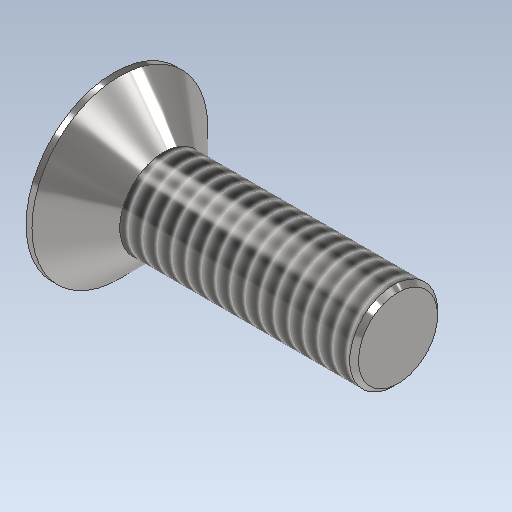
# Autodesk Inventor part: ネジ皿M3L8
Saved by Autodesk Inventor 2020.2 (Build 242310000, 310)
## iProperties
Created: 2020-04-20
Part Number: ネジ皿M3L8
Material: 鋼、高強度、低合金
Document SubType Name: Modeling
Designer: aoyama
Density: 7.85 g/cm^3
Appearance: 鋼 - つや出し
Mass: 0.649002 g
Surface Area: 1.51758 cm^2
Volume: 0.0826754 cm^3
Author: aoyama
Autodesk Inventor part; units mm, degrees
ref_plane "YZ Plane" through (0, 0, 0) normal (1, 0, 0) x (0, 1, 0)
ref_plane "XZ Plane" through (0, 0, 0) normal (0, 1, 0) x (-1, 0, 0)
ref_plane "XY Plane" through (0, 0, 0) normal (0, 0, 1) x (1, 0, 0)
sketch "スケッチ1" plane through (0, 0, 0) normal (0, 0, 1) x (1, 0, 0)
  line L0 (0, 0) -> (0, 3)
  line L1 (0, 3) -> (0.2, 3)
  line L2 (0.2, 3) -> (1.7, 1.5)
  line L3 (1.7, 1.5) -> (9.7, 1.5)
  line L4 (9.7, 1.5) -> (9.7, 0)
  line L5 (0, 0) -> (9.7, 0)
  dimension "d0" = 45
  dimension "d1" = 3
  dimension "d2" = 1.7
  dimension "d3" = 1.5
  dimension "d4" = 8
  constraints: 12 end point, 3 horizontal, 2 vertical
  measures "d0" angle of L0 L2
  measures "d1" distance of L0.start L0.end
  measures "d2" distance from line of L0 L2.end
  measures "d3" distance between parallel lines of L3 L5
  measures "d4" distance of L3.end L2.end
revolve "回転1" add sketch "スケッチ1" angle 360 about axis through (0, 0, 0) along (1, 0, 0)
thread "ねじ1" size "M3x0.5" class "6g" standard "ANSI Metric M Profile" length 44.8
sketch "スケッチ2" plane through (0, 0, 0) normal (-1, 0, 0) x (0, 0, 1)
  line L0 (0.5774, 1) -> (1.1547, 0)
  line L1 (1.1547, 0) -> (0.5774, -1)
  line L2 (0.5774, -1) -> (-0.5774, -1)
  line L3 (-0.5774, -1) -> (-1.1547, 0)
  line L4 (-1.1547, 0) -> (-0.5774, 1)
  line L5 (-0.5774, 1) -> (0.5774, 1)
  circle A0 centre (0, 0) radius 1.1547
  point P0 (0, 0)
  point P1 (0, 0)
  dimension "d8" = 2
  constraints: 12 end point, 1 coincident, 1 horizontal, 16 other
  measures "d8" distance between parallel lines of L2 L5
extrude "押し出し1" cut sketch "スケッチ2" against normal blind 1.2 contours L0 L1 L2 L3 L4 L5
chamfer "面取り1" distance 0.05 angle 45 6 edges at (0, -0.5, -0.866) (0, 0.5, -0.866) (0, 1, 0) (0, 0.5, 0.866) (0, -1, 0) (0, -0.5, 0.866)
chamfer "面取り2" distance 0.15 angle 45 1 edges at (9.7, -1.5, 0)
